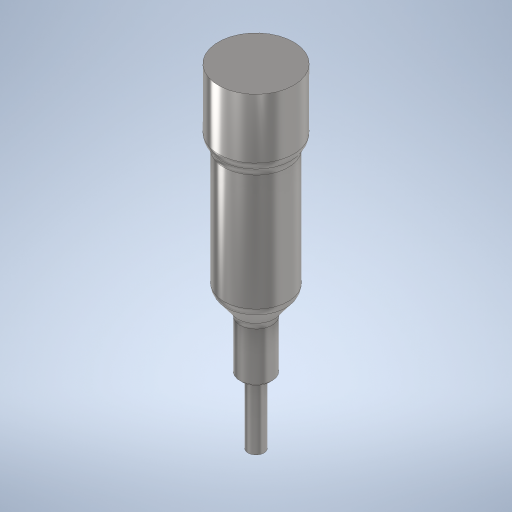
# Autodesk Inventor part: screwdriver
Saved by Autodesk Inventor 2024.3 (Build 283343000, 343)
## iProperties
Created: 2025-07-30
Part Number: screwdriver
Material: Acciaio inossidabile
Document SubType Name: Modeling
Designer: chris
Density: 8 g/cm^3
Appearance: Semilucidato
Author: chris
Autodesk Inventor part; units mm, degrees
ref_plane "YZ Plane" through (0, 0, 0) normal (1, 0, 0) x (0, 1, 0)
ref_plane "XZ Plane" through (0, 0, 0) normal (0, 1, 0) x (-1, 0, 0)
ref_plane "XY Plane" through (0, 0, 0) normal (0, 0, 1) x (1, 0, 0)
sketch "Schizzo1" plane through (0, 0, 0) normal (0, 0, 1) x (1, 0, 0)
  circle A0 centre (0, 0) radius 0.035
  dimension "d0" = 0.07
  constraints: 1 centre point, 1 coincident
  measures "d0" diameter of A0
extrude "Estrusione1" add sketch "Schizzo1" along normal blind 0.06
sketch "Schizzo2" plane through (0, 0, 0.06) normal (0, 0, 1) x (1, 0, 0)
  circle A0 centre (0, 0) radius 0.03
  dimension "d3" = 0.06
  constraints: 1 centre point, 1 coincident
  measures "d3" diameter of A0
extrude "Estrusione2" add sketch "Schizzo2" along normal blind 0.12
sketch "Schizzo3" plane through (0, 0, 0) normal (1, 0, 0) x (0, 1, 0)
  line L0 (0.03, 0.18) -> (-0.03, 0.18) construction
  line L1 (-0.03, 0.06) -> (0.03, 0.06) construction
  line L2 (0, 0) -> (0, 0.2309)
  line L3 (0.03, 0.18) -> (0.015, 0.2)
  line L4 (0.015, 0.2) -> (0, 0.2)
  line L5 (0, 0.2) -> (0, 0.18)
  line L6 (0.03, 0.18) -> (0, 0.18)
  dimension "d6" = 0.02
  dimension "d7" = 0.015
  constraints: 10 end point, 2 perpendicular, 2 point on line, 1 collinear, 1 midpoint
  measures "d6" distance from line of L4 L0.start
  measures "d7" distance of L3.end L4.end
revolve "Rivoluzione1" add sketch "Schizzo3" angle 360 about axis through (0, 0, 0) along (0, 0, 1)
sketch "Schizzo4" plane through (0, 0, 0.2) normal (0, 0, 1) x (1, 0, 0)
  circle A0 centre (0, 0) radius 0.015 projected
extrude "Estrusione3" add sketch "Schizzo4" along normal blind 0.05
sketch "Schizzo5" plane through (0, 0, 0.25) normal (0, 0, 1) x (1, 0, 0)
  circle A0 centre (0, 0) radius 0.0075
  dimension "d11" = 0.015
  constraints: 1 centre point, 1 coincident
  measures "d11" diameter of A0
extrude "Estrusione4" add sketch "Schizzo5" along normal blind 0.06
fillet "Raccordo1" radius 0.01 1 edges at (-0.03, 0, 0.06)
chamfer "Smusso1" distance 0.002 angle 45 1 edges at (-0.015, 0, 0.25)
fillet "Raccordo2" radius 0.01 4 edges at (-0.0106, -0.0106, 0.2) (0.0106, 0.0106, 0.2) (0.0212, 0.0212, 0.18) (-0.0212, -0.0212, 0.18)
fillet "Raccordo3" radius 0.01 1 edges at (-0.035, 0, 0.06)
